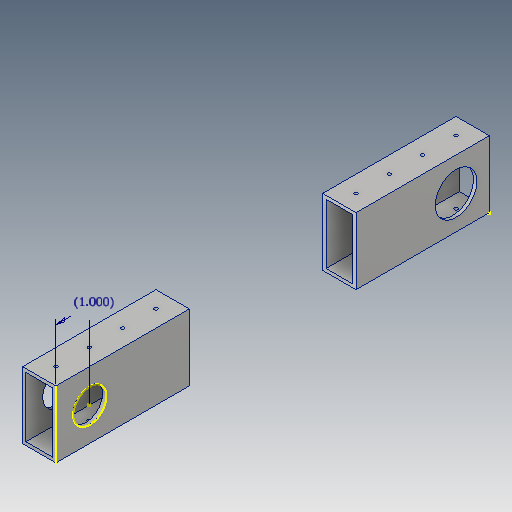
# Autodesk Inventor part: Support Pivs 252
Saved by Autodesk Inventor 2018 (Build 220112000, 112)
## iProperties
Created: 2018-01-08
Part Number: Support Pivs 252
Material: Aluminum 6061
Document SubType Name: Modeling
Designer: dsayers
Density: 2.7 g/cm^3
Appearance: Aluminum - Flat
Mass: 194.187 g
Surface Area: 588.056 cm^2
Volume: 71.9211 cm^3
Author: dsayers
Autodesk Inventor part; units mm, degrees
ref_plane "YZ Plane" through (0, 0, 0) normal (1, 0, 0) x (0, 1, 0)
ref_plane "XZ Plane" through (0, 0, 0) normal (0, 1, 0) x (-1, 0, 0)
ref_plane "XY Plane" through (0, 0, 0) normal (0, 0, 1) x (1, 0, 0)
sketch "Sketch1" plane through (0, 0, 0) normal (0, 0, 1) x (1, 0, 0)
  line L0 (0, 0) -> (25.4, 0)
  line L1 (25.4, 0) -> (25.4, 50.8)
  line L2 (25.4, 50.8) -> (0, 50.8)
  line L3 (0, 50.8) -> (0, 0)
  dimension "d0" = 25.4
  dimension "d1" = 50.8
  constraints: 8 end point, 2 parallel, 1 horizontal, 1 perpendicular
  measures "d0" distance of L1.end L2.end
  measures "d1" distance of L0.end L1.end
extrude "Extrusion1" add sketch "Sketch1" along normal blind 330.2
shell "Shell1" thickness 2.54 removed faces 2 at (8.4667, 33.8667, 0) at (8.4667, 33.8667, 330.2)
sketch "Sketch2" plane through (0, 50.8, 0) normal (0, 1, 0) x (1, 0, 0)
  line L0 (25.4, 0) -> (0, 0) projected
  line L1 (0, 0) -> (0, -330.2) projected
  point P0 (12.7, -12.7)
  point P1 (12.7, -38.1)
  point P2 (12.7, -63.5)
  point P3 (12.7, -88.9)
  point P4 (12.7, -114.3)
  point P5 (12.7, -139.7)
  point P6 (12.7, -165.1)
  point P7 (12.7, -190.5)
  point P8 (12.7, -215.9)
  point P9 (12.7, -241.3)
  point P10 (12.7, -266.7)
  point P11 (12.7, -292.1)
  point P12 (12.7, -317.5)
  point P13 (12.7, -342.9)
  point P14 (12.7, -368.3)
  point P15 (12.7, -393.7)
  point P16 (12.7, -419.1)
  point P17 (12.7, -444.5)
  point P18 (12.7, -469.9)
  point P19 (12.7, -495.3)
  point P20 (12.7, -520.7)
  point P21 (12.7, -546.1)
  point P22 (12.7, -571.5)
  point P23 (12.7, -596.9)
  point P24 (12.7, -622.3)
  point P25 (12.7, -647.7)
  point P26 (12.7, -673.1)
  point P27 (12.7, -698.5)
  point P28 (12.7, -723.9)
  point P29 (12.7, -749.3)
  point P30 (12.7, -774.7)
  point P31 (12.7, -800.1)
  point P32 (12.7, -825.5)
  point P33 (12.7, -850.9)
  point P34 (12.7, -876.3)
  point P35 (12.7, -901.7)
  point P36 (12.7, -927.1)
  dimension "d5" = 12.7
  dimension "d6" = 12.7
  dimension "d9" = 25.4
  constraints: 1 vertical, 36 other
  measures "d5" distance from line of L0 point (12.7, -12.7)
  measures "d6" distance from line of L1 point (12.7, -12.7)
  measures "d9" distance of point (12.7, -12.7) point (12.7, -38.1)
hole "Hole1" at (12.7, 50.8, 12.7) at (12.7, 50.8, 38.1) at (12.7, 50.8, 63.5) at (12.7, 50.8, 88.9) at (12.7, 50.8, 114.3) at (12.7, 50.8, 139.7) at (12.7, 50.8, 165.1) at (12.7, 50.8, 190.5) at (12.7, 50.8, 215.9) at (12.7, 50.8, 241.3) at (12.7, 50.8, 266.7) at (12.7, 50.8, 292.1) at (12.7, 50.8, 317.5) at (12.7, 50.8, 342.9) at (12.7, 50.8, 368.3) at (12.7, 50.8, 393.7) at (12.7, 50.8, 419.1) at (12.7, 50.8, 444.5) at (12.7, 50.8, 469.9) at (12.7, 50.8, 495.3) at (12.7, 50.8, 520.7) at (12.7, 50.8, 546.1) at (12.7, 50.8, 571.5) at (12.7, 50.8, 596.9) at (12.7, 50.8, 622.3) at (12.7, 50.8, 647.7) at (12.7, 50.8, 673.1) at (12.7, 50.8, 698.5) at (12.7, 50.8, 723.9) at (12.7, 50.8, 749.3) at (12.7, 50.8, 774.7) at (12.7, 50.8, 800.1) at (12.7, 50.8, 825.5) at (12.7, 50.8, 850.9) at (12.7, 50.8, 876.3) at (12.7, 50.8, 901.7) direction (0, -1, 0) diameter 2.54 depth 50.8 tip angle 118
sketch "Sketch10" plane through (25.4, 0, 0) normal (1, 0, 0) x (0, 0, -1)
  line L0 (0, 50.8) -> (-330.2, 50.8) projected
  line L1 (0, 0) -> (0, 50.8) projected
  line L2 (-330.2, 0) -> (-330.2, 50.8) projected
  point P0 (-25.4, 25.4)
  point P1 (-304.8, 25.4)
  dimension "d66" = 25.4
  dimension "d67" = 25.4
  dimension "d68" = 279.4
  dimension "d69" = 25.4
  dimension "d70" = 25.4
  measures "d66" distance from line of L0 point (-304.8, 25.4)
  measures "d67" distance from line of L0 point (-25.4, 25.4)
  measures "d68" distance of point (-304.8, 25.4) point (-25.4, 25.4)
  measures "d69" distance from line of L1 point (-25.4, 25.4)
  measures "d70" distance from line of L2 point (-304.8, 25.4)
hole "Hole5" at (25.4, 25.4, 25.4) at (25.4, 25.4, 304.8) direction (-1, 0, 0) diameter 12.7 depth 25.4 tip angle 118
sketch "Sketch11" plane through (25.4, 0, 0) normal (1, 0, 0) x (0, 0, -1)
  line L0 (0, 50.8) -> (-330.2, 50.8) projected
  line L1 (0, 0) -> (-330.2, 0) projected
  line L2 (-228.6, 50.8) -> (-101.6, 50.8)
  line L3 (-101.6, 50.8) -> (-101.6, 0)
  line L4 (-101.6, 0) -> (-228.6, 0)
  line L5 (-228.6, 0) -> (-228.6, 50.8)
  line L6 (0, 0) -> (0, 50.8) projected
  line L7 (-330.2, 0) -> (-330.2, 50.8) projected
  dimension "d78" = 101.6
  dimension "d79" = 101.6
  constraints: 8 end point, 2 parallel, 2 point on line, 1 horizontal, 1 perpendicular
  measures "d78" distance between parallel lines of L6 L3
  measures "d79" distance between parallel lines of L7 L5
extrude "Extrusion6" cut sketch "Sketch11" against normal blind 25.4 contours L3 L1 L5 L0
sketch "Sketch12" plane through (25.4, 0, 0) normal (1, 0, 0) x (0, 0, -1)
  circle A0 centre (-25.4, 25.4) radius 6.35 projected
  circle A1 centre (-25.4, 25.4) radius 6.35 projected
  circle A2 centre (-25.4, 25.4) radius 15.875
  circle A3 centre (-25.4, 25.4) radius 9.525
  line L0 (-35.3561, 30.0738) -> (-26.3304, 36.3591)
  line L1 (-26.3304, 36.3591) -> (-16.3743, 31.6853)
  line L2 (-16.3743, 31.6853) -> (-15.4439, 20.7262)
  line L3 (-15.4439, 20.7262) -> (-24.4696, 14.4409)
  line L4 (-24.4696, 14.4409) -> (-34.4257, 19.1147)
  line L5 (-34.4257, 19.1147) -> (-35.3561, 30.0738)
  point P0 (0, 0)
  dimension "d82" = 31.75
  dimension "d83" = 19.05
  dimension "d84" = 19.05
  constraints: 12 end point, 3 coincident, 2 centre point, 13 other
  measures "d82" diameter of A2
  measures "d83" diameter of A3
  measures "d84" distance between parallel lines of L2 L5
extrude "Extrusion7" cut sketch "Sketch12" against normal blind 25.4 contours A0 | A2 | A3 | A3 L2 L3 | A3 L1 L2 | L3 L4 A3 | A3 L0 L1 | L4 L5 A3 | A3 L5 L0
sketch "Sketch13" plane through (25.4, 0, 330.2) normal (1, 0, 0) x (0, 0, -1)
  line L0 (101.6, 50.8) -> (0, 50.8) projected
  line L1 (101.6, 0) -> (101.6, 50.8) projected
  line L2 (101.6, 50.8) -> (0, 50.8) projected
  line L3 (0, 0) -> (0, 50.8) projected
  line L4 (101.6, 0) -> (0, 0) projected
  circle A0 centre (25.4, 25.4) radius 6.35 projected
  circle A1 centre (25.4, 25.4) radius 12.7
  point P0 (330.2, 0)
  dimension "d87" = 25.4
  constraints: 1 centre point, 1 coincident
  measures "d87" diameter of A1
extrude "Extrusion8" cut sketch "Sketch13" against normal blind 25.4 contours A1
sketch "Sketch14" plane through (25.4, 0, 330.2) normal (1, 0, 0) x (0, 0, -1)
  circle A0 centre (25.4, 25.4) radius 12.7 projected
  line L0 (0, 0) -> (0, 50.8) projected
  point P0 (330.2, 0)
  dimension "d90" = 25.4
  measures "d90" distance from line of L0 A0.centre
equation "\"d69\" = d70"
body "Solid1"
